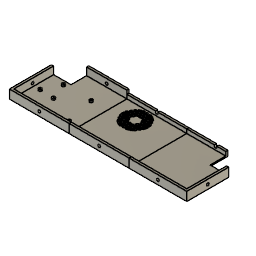
XY_Plotter_Main_Body (Autodesk Fusion 360 archive; units mm, degrees)
design "main board"
Autodesk Fusion 360 part; units mm, degrees
sketch "Sketch1" plane through (0, 0, 0) normal (0, 0, 1) x (1, 0, 0)
  line L0 (50, 35) -> (-50, 35)
  line L1 (-50, 35) -> (-50, -35)
  line L2 (-50, -35) -> (50, -35)
  line L3 (50, -35) -> (50, 35)
  line L4 (50, 35) -> (-50, -35) construction
  line L5 (-50, 35) -> (50, -35) construction
  line L6 (50, 34) -> (-50, 34) construction
  line L7 (34, -35) -> (34, 35) construction
  line L8 (-32, 35) -> (-32, -35) construction
  circle A0 centre (-30.25, 32.25) radius 1.75
  circle A1 centre (32.25, 32.25) radius 1.75
  line L9 (-49, 35) -> (-49, -35) construction
  line L10 (-50, -5) -> (50, -5) construction
  circle A2 centre (-47.25, -3.25) radius 1.75
  line L11 (-50, -34) -> (50, -34) construction
  line L12 (49, -35) -> (49, 35) construction
  circle A3 centre (47.25, -32.25) radius 1.75
  line L13 (-50, -7) -> (50, -7) construction
  line L14 (-17, 35) -> (-17, -35) construction
  circle A4 centre (-15.25, -5.25) radius 1.75
  line L15 (67.5, 67.5) -> (-67.5, 67.5)
  line L16 (-67.5, 67.5) -> (-67.5, -67.5)
  line L17 (-67.5, -67.5) -> (67.5, -67.5)
  line L18 (67.5, -67.5) -> (67.5, 67.5)
  line L19 (67.5, 67.5) -> (-67.5, -67.5) construction
  line L20 (-67.5, 67.5) -> (67.5, -67.5) construction
  dimension "d1" = 100
  dimension "d2" = 70
  dimension "d3" = -1
  dimension "d4" = -16
  dimension "d5" = -18
  dimension "d6" = 1.75
  dimension "d7" = 1.75
  dimension "d8" = -1
  dimension "d9" = -30
  dimension "d10" = 1.75
  dimension "d11" = -1
  dimension "d12" = -1
  dimension "d13" = 1.75
  dimension "d14" = -28
  dimension "d15" = -33
  dimension "d16" = 1.75
  dimension "d19" = 135
  dimension "d20" = 135
  constraint horizontal L0
  constraint perpendicular L0 L1
  constraint parallel L0 L2
  constraint parallel L1 L3
  constraint coincident L4 origin
  constraint coincident L5 origin
  constraint tangent L8 A0
  constraint tangent L6 A0
  constraint tangent L7 A1
  constraint tangent L6 A1
  constraint tangent L10 A2
  constraint tangent L9 A2
  constraint tangent L12 A3
  constraint tangent L11 A3
  constraint tangent L13 A4
  constraint tangent L14 A4
  constraint horizontal L15
  constraint perpendicular L15 L16
  constraint parallel L15 L17
  constraint parallel L16 L18
  constraint coincident L19 origin
  constraint coincident L20 origin
  measures "d1" distance of L1.end L2.end
  measures "d2" distance of L0.end L1.end
  measures "d6" radius of A0
  measures "d7" radius of A1
  measures "d10" radius of A2
  measures "d13" radius of A3
  measures "d16" radius of A4
  measures "d19" distance of L16.end L17.end
  measures "d20" distance of L15.end L16.end
extrude "Extrude1" add sketch "Sketch1" along normal blind 2 contours L0 L1 L2 L3 makes body 1
sketch "Sketch2" plane through (0, 0, 2) normal (0, 0, 1) x (-1, 0, 0)
  circle A0 centre (47.25, 3.25) radius 1.75
  circle A1 centre (30.25, -32.25) radius 1.75
  circle A2 centre (15.25, 5.25) radius 1.75
  circle A3 centre (-47.25, 32.25) radius 1.75
  circle A4 centre (-32.25, -32.25) radius 1.75
  line L0 (-50, 35) -> (-50, -35)
  line L1 (-50, -35) -> (50, -35)
  line L2 (50, -35) -> (50, 35)
  line L3 (50, 35) -> (-50, 35)
  line L4 (0, 0) -> (0, -15)
  line L5 (-67.5, -82.5) -> (67.5, -82.5)
  line L6 (67.5, -82.5) -> (67.5, 52.5)
  line L7 (67.5, 52.5) -> (-67.5, 52.5)
  line L8 (-67.5, 52.5) -> (-67.5, -82.5)
  line L9 (-67.5, -82.5) -> (67.5, 52.5) construction
  line L10 (67.5, -82.5) -> (-67.5, 52.5) construction
  line L11 (-67.5, -77.5) -> (62.5, -77.5)
  line L12 (62.5, -77.5) -> (62.5, 52.5)
  line L13 (67.5, -82.5) -> (23.5, -82.5)
  line L14 (23.5, -82.5) -> (23.5, -42.5)
  line L15 (23.5, -42.5) -> (67.5, -42.5)
  line L16 (67.5, -42.5) -> (67.5, -82.5)
  line L17 (67.5, 47.5) -> (-67.5, 47.5)
  point P0 (0, -15)
  dimension "d21" = 15
  dimension "d22" = 135
  dimension "d23" = 135
  dimension "d24" = -5
  dimension "d25" = 44
  dimension "d26" = 40
  dimension "d37" = -5
  constraint coincident L4.start origin
  constraint vertical L4
  constraint horizontal L5
  constraint perpendicular L5 L6
  constraint parallel L5 L7
  constraint parallel L6 L8
  constraint coincident L9 P0
  constraint coincident L10 P0
  constraint coincident P0 L4.end
  constraint horizontal L13
  constraint vertical L14
  constraint horizontal L15
  constraint vertical L16
  measures "d21" distance of L4.start P0
  measures "d22" distance of L6.end L7.end
  measures "d23" distance of L5.end L6.end
  measures "d25" distance of L5.end L13.end
  measures "d26" distance of L5.end L15.end
extrude "Extrude2" add sketch "Sketch2" against normal blind 3 from surface at -2 separate body contours L0 L1 L2 L3 | L5 L8 L11 L14 | L8 L11 L12 L14 L15 L17 | L7 L8 L12 L17 | L6 L12 L15 L17 | L6 L7 L12 L17 makes body 2
extrude "Extrude3" add sketch "Sketch2" along normal blind 15 and the other way blind 2 contours L5 L8 L11 L14 | L7 L8 L12 L17 | L6 L12 L15 L17 | L6 L7 L12 L17 bodies 2
sketch "Sketch3" plane through (0, 0, 0) normal (0, 0, 1) x (-1, 0, 0)
  line L0 (-67.5, -77.5) -> (23.5, -77.5)
  line L1 (23.5, -77.5) -> (23.5, -42.5)
  line L2 (23.5, -42.5) -> (62.5, -42.5)
  line L3 (62.5, -42.5) -> (62.5, 47.5)
  line L4 (62.5, 47.5) -> (-67.5, 47.5)
  line L5 (-67.5, 47.5) -> (-67.5, -77.5)
  circle A0 centre (47.25, 3.25) radius 1.75
  circle A1 centre (15.25, 5.25) radius 1.75
  circle A2 centre (30.25, -32.25) radius 1.75
  circle A3 centre (-47.25, 32.25) radius 1.75
  circle A4 centre (-32.25, -32.25) radius 1.75
  circle A5 centre (30.25, -32.25) radius 3.5
  circle A6 centre (-32.25, -32.25) radius 3.5
  circle A7 centre (-47.25, 32.25) radius 3.5
  circle A8 centre (15.25, 5.25) radius 3.5
  circle A9 centre (47.25, 3.25) radius 3.5
  circle A10 centre (15.25, 5.25) radius 1.25
  circle A11 centre (47.25, 3.25) radius 1.25
  circle A12 centre (30.25, -32.25) radius 1.25
  circle A13 centre (-32.25, -32.25) radius 1.25
  circle A14 centre (-47.25, 32.25) radius 1.25
  dimension "d38" = 7
  dimension "d39" = 7
  dimension "d40" = 7
  dimension "d41" = 7
  dimension "d42" = 7
  dimension "d43" = 2.5
  dimension "d44" = 2.5
  dimension "d45" = 2.5
  dimension "d46" = 2.5
  dimension "d47" = 2.5
  constraint concentric A2 A5
  constraint concentric A4 A6
  constraint concentric A3 A7
  constraint concentric A1 A8
  constraint concentric A0 A9
  constraint concentric A1 A10
  constraint concentric A0 A11
  constraint concentric A2 A12
  constraint concentric A4 A13
  constraint concentric A3 A14
  measures "d38" diameter of A5
  measures "d39" diameter of A6
  measures "d40" diameter of A7
  measures "d41" diameter of A8
  measures "d42" diameter of A9
  measures "d43" diameter of A10
  measures "d44" diameter of A11
  measures "d45" diameter of A12
  measures "d46" diameter of A13
  measures "d47" diameter of A14
extrude "Extrude5" add sketch "Sketch3" against normal blind 3 contours A0 | A1 | A2 | A3 | A4 bodies 2
extrude "Extrude6" add sketch "Sketch3" along normal blind 3 contours A0 | A1 | A2 | A3 | A4 | A5 | A6 | A7 | A8 | A9 bodies 2
move_body "Move1" bodies 1 to x (1, 0, 0) y (0, 1, 0) z (0, 0, 1) at (0, 0, 3)
sketch "Sketch4" plane through (0, -52.5, 0) normal (0, -1, 0) x (1, 0, 0)
  line L0 (-67.5, 17) -> (-67.5, -3)
  line L1 (-67.5, -3) -> (67.5, -3)
  line L2 (67.5, -3) -> (67.5, 17)
  line L3 (67.5, 17) -> (-67.5, 17)
  line L4 (0, 17) -> (0, -3)
  circle A0 centre (0, 7) radius 3
  circle A1 centre (0, 7) radius 4.5
  dimension "d52" = 6
  dimension "d53" = 9
  constraint midpoint L3 L4.start
  constraint midpoint L1 L4.end
  constraint midpoint L4 A0.centre
  constraint concentric A0 A1
  measures "d52" diameter of A0
  measures "d53" diameter of A1
extrude "Extrude7" cut sketch "Sketch4" against normal blind 5 contours L4 A0 | L4 A0 bodies 2
sketch "Sketch5" plane through (0, 82.5, 0) normal (0, 1, 0) x (-1, 0, 0)
  line L0 (-67.5, 17) -> (-67.5, -3)
  line L1 (-67.5, -3) -> (23.5, -3)
  line L2 (23.5, -3) -> (23.5, 17)
  line L3 (23.5, 17) -> (-67.5, 17)
  line L4 (-22, 17) -> (-22, -3) construction
  circle A0 centre (-22, 7) radius 3
  dimension "d56" = 6
  constraint midpoint L3 L4.start
  constraint midpoint L1 L4.end
  constraint midpoint L4 A0.centre
  measures "d56" diameter of A0
extrude "Extrude8" cut sketch "Sketch5" against normal blind 5 contours A0 bodies 2
sketch "Sketch6" plane through (-67.5, 0, 0) normal (-1, 0, 0) x (0, -1, 0)
  line L0 (-42.5, 17) -> (-42.5, -3)
  line L1 (-42.5, -3) -> (52.5, -3)
  line L2 (52.5, -3) -> (52.5, 17)
  line L3 (52.5, 17) -> (-42.5, 17)
  line L4 (5, 17) -> (5, -3) construction
  circle A0 centre (5, 7) radius 3
  dimension "d59" = 6
  constraint midpoint L3 L4.start
  constraint midpoint L1 L4.end
  constraint midpoint L4 A0.centre
  measures "d59" diameter of A0
extrude "Extrude9" cut sketch "Sketch6" against normal blind 5 contours A0 bodies 2
extrude "Extrude10" add 1 faces at (67.5, -50.8333, 4.6667) along direction (1, 0, 0) blind 135 separate body on bodies 2 makes body 3
extrude "Extrude11" cut 1 faces at (112.5, 79.1667, 17) along direction (0, 0, -1) blind 8 on bodies 3 bodies 3
sketch "Sketch7" plane through (0, -52.5, 0) normal (0, -1, 0) x (1, 0, 0)
  line L0 (67.5, 17) -> (67.5, -3)
  line L1 (67.5, -3) -> (202.5, -3)
  line L2 (202.5, -3) -> (202.5, 17)
  line L3 (202.5, 17) -> (67.5, 17)
  line L4 (135, 17) -> (135, -3) construction
  circle A0 centre (135, 7) radius 3
  dimension "d66" = 6
  constraint midpoint L3 L4.start
  constraint midpoint L1 L4.end
  constraint midpoint L4 A0.centre
  measures "d66" diameter of A0
extrude "Extrude12" cut sketch "Sketch7" against normal blind 135 contours A0 bodies 3
sketch "Sketch8" plane through (0, 0, -3) normal (0, 0, -1) x (1, 0, 0)
  line L0 (67.5, 52.5) -> (67.5, -82.5)
  line L1 (67.5, -82.5) -> (202.5, -82.5)
  line L2 (202.5, -82.5) -> (202.5, 52.5)
  line L3 (202.5, 52.5) -> (67.5, 52.5)
  line L4 (89.5, 52.5) -> (89.5, -82.5)
  line L5 (67.5, -74.5) -> (202.5, -74.5)
  circle A0 centre (118.5, -45.5) radius 29
  circle A1 centre (118.5, -45.5) radius 10
  line L6 (118.5, -45.5) -> (108.5, -45.5)
  line L7 (108.5, -45.5) -> (89.5, -45.5) construction
  line L8 (115.5, -47.2321) -> (118.5, -48.9641)
  line L9 (118.5, -48.9641) -> (121.5, -47.2321)
  line L10 (121.5, -47.2321) -> (121.5, -43.7679)
  line L11 (121.5, -43.7679) -> (118.5, -42.0359)
  line L12 (118.5, -42.0359) -> (115.5, -43.7679)
  line L13 (115.5, -43.7679) -> (115.5, -47.2321)
  line L14 (118.5, -45.5) -> (117, -48.0981)
  line L15 (118.5, -45.5) -> (120, -48.0981)
  line L16 (115.5, 2.9974) -> (118.5, 1.2654)
  line L17 (118.5, 1.2654) -> (121.5, 2.9974)
  line L18 (121.5, 2.9974) -> (121.5, 6.4615)
  line L19 (121.5, 6.4615) -> (118.5, 8.1936)
  line L20 (118.5, 8.1936) -> (115.5, 6.4615)
  line L21 (115.5, 6.4615) -> (115.5, 2.9974)
  line L22 (119.125, -3.2813) -> (122.125, -5.0133)
  line L23 (122.125, -5.0133) -> (125.125, -3.2813)
  line L24 (125.125, -3.2813) -> (125.125, 0.1828)
  line L25 (125.125, 0.1828) -> (122.125, 1.9149)
  line L26 (122.125, 1.9149) -> (119.125, 0.1828)
  line L27 (119.125, 0.1828) -> (119.125, -3.2813)
  line L28 (122.75, -9.5599) -> (125.75, -11.292)
  line L29 (125.75, -11.292) -> (128.75, -9.5599)
  line L30 (128.75, -9.5599) -> (128.75, -6.0958)
  line L31 (128.75, -6.0958) -> (125.75, -4.3638)
  line L32 (125.75, -4.3638) -> (122.75, -6.0958)
  line L33 (122.75, -6.0958) -> (122.75, -9.5599)
  line L34 (126.375, -15.8386) -> (129.375, -17.5707)
  line L35 (129.375, -17.5707) -> (132.375, -15.8386)
  line L36 (132.375, -15.8386) -> (132.375, -12.3745)
  line L37 (132.375, -12.3745) -> (129.375, -10.6425)
  line L38 (129.375, -10.6425) -> (126.375, -12.3745)
  line L39 (126.375, -12.3745) -> (126.375, -15.8386)
  line L40 (130, -22.1173) -> (133, -23.8494)
  line L41 (133, -23.8494) -> (136, -22.1173)
  line L42 (136, -22.1173) -> (136, -18.6532)
  line L43 (136, -18.6532) -> (133, -16.9212)
  line L44 (133, -16.9212) -> (130, -18.6532)
  line L45 (130, -18.6532) -> (130, -22.1173)
  line L46 (133.625, -28.396) -> (136.625, -30.128)
  line L47 (136.625, -30.128) -> (139.625, -28.396)
  line L48 (139.625, -28.396) -> (139.625, -24.9319)
  line L49 (139.625, -24.9319) -> (136.625, -23.1998)
  line L50 (136.625, -23.1998) -> (133.625, -24.9319)
  line L51 (133.625, -24.9319) -> (133.625, -28.396)
  line L52 (137.25, -34.6747) -> (140.25, -36.4067)
  line L53 (140.25, -36.4067) -> (143.25, -34.6747)
  line L54 (143.25, -34.6747) -> (143.25, -31.2106)
  line L55 (143.25, -31.2106) -> (140.25, -29.4785)
  line L56 (140.25, -29.4785) -> (137.25, -31.2106)
  line L57 (137.25, -31.2106) -> (137.25, -34.6747)
  line L58 (140.875, -40.9534) -> (143.875, -42.6854)
  line L59 (143.875, -42.6854) -> (146.875, -40.9534)
  line L60 (146.875, -40.9534) -> (146.875, -37.4893)
  line L61 (146.875, -37.4893) -> (143.875, -35.7572)
  line L62 (143.875, -35.7572) -> (140.875, -37.4893)
  line L63 (140.875, -37.4893) -> (140.875, -40.9534)
  line L64 (144.5, -47.2321) -> (147.5, -48.9641)
  line L65 (147.5, -48.9641) -> (150.5, -47.2321)
  line L66 (150.5, -47.2321) -> (150.5, -43.7679)
  line L67 (150.5, -43.7679) -> (147.5, -42.0359)
  line L68 (147.5, -42.0359) -> (144.5, -43.7679)
  line L69 (144.5, -43.7679) -> (144.5, -47.2321)
  line L70 (111.875, -3.2813) -> (114.875, -5.0133)
  line L71 (114.875, -5.0133) -> (117.875, -3.2813)
  line L72 (117.875, -3.2813) -> (117.875, 0.1828)
  line L73 (117.875, 0.1828) -> (114.875, 1.9149)
  line L74 (114.875, 1.9149) -> (111.875, 0.1828)
  line L75 (111.875, 0.1828) -> (111.875, -3.2813)
  line L76 (115.5, -9.5599) -> (118.5, -11.292)
  line L77 (118.5, -11.292) -> (121.5, -9.5599)
  line L78 (121.5, -9.5599) -> (121.5, -6.0958)
  line L79 (121.5, -6.0958) -> (118.5, -4.3638)
  line L80 (118.5, -4.3638) -> (115.5, -6.0958)
  line L81 (115.5, -6.0958) -> (115.5, -9.5599)
  line L82 (119.125, -15.8386) -> (122.125, -17.5707)
  line L83 (122.125, -17.5707) -> (125.125, -15.8386)
  line L84 (125.125, -15.8386) -> (125.125, -12.3745)
  line L85 (125.125, -12.3745) -> (122.125, -10.6425)
  line L86 (122.125, -10.6425) -> (119.125, -12.3745)
  line L87 (119.125, -12.3745) -> (119.125, -15.8386)
  line L88 (122.75, -22.1173) -> (125.75, -23.8494)
  line L89 (125.75, -23.8494) -> (128.75, -22.1173)
  line L90 (128.75, -22.1173) -> (128.75, -18.6532)
  line L91 (128.75, -18.6532) -> (125.75, -16.9212)
  line L92 (125.75, -16.9212) -> (122.75, -18.6532)
  line L93 (122.75, -18.6532) -> (122.75, -22.1173)
  line L94 (126.375, -28.396) -> (129.375, -30.128)
  line L95 (129.375, -30.128) -> (132.375, -28.396)
  line L96 (132.375, -28.396) -> (132.375, -24.9319)
  line L97 (132.375, -24.9319) -> (129.375, -23.1998)
  line L98 (129.375, -23.1998) -> (126.375, -24.9319)
  line L99 (126.375, -24.9319) -> (126.375, -28.396)
  line L100 (130, -34.6747) -> (133, -36.4067)
  line L101 (133, -36.4067) -> (136, -34.6747)
  line L102 (136, -34.6747) -> (136, -31.2106)
  line L103 (136, -31.2106) -> (133, -29.4785)
  line L104 (133, -29.4785) -> (130, -31.2106)
  line L105 (130, -31.2106) -> (130, -34.6747)
  line L106 (133.625, -40.9534) -> (136.625, -42.6854)
  line L107 (136.625, -42.6854) -> (139.625, -40.9534)
  line L108 (139.625, -40.9534) -> (139.625, -37.4893)
  line L109 (139.625, -37.4893) -> (136.625, -35.7572)
  line L110 (136.625, -35.7572) -> (133.625, -37.4893)
  line L111 (133.625, -37.4893) -> (133.625, -40.9534)
  line L112 (137.25, -47.2321) -> (140.25, -48.9641)
  line L113 (140.25, -48.9641) -> (143.25, -47.2321)
  line L114 (143.25, -47.2321) -> (143.25, -43.7679)
  line L115 (143.25, -43.7679) -> (140.25, -42.0359)
  line L116 (140.25, -42.0359) -> (137.25, -43.7679)
  line L117 (137.25, -43.7679) -> (137.25, -47.2321)
  line L118 (140.875, -53.5107) -> (143.875, -55.2428)
  line L119 (143.875, -55.2428) -> (146.875, -53.5107)
  line L120 (146.875, -53.5107) -> (146.875, -50.0466)
  line L121 (146.875, -50.0466) -> (143.875, -48.3146)
  line L122 (143.875, -48.3146) -> (140.875, -50.0466)
  line L123 (140.875, -50.0466) -> (140.875, -53.5107)
  line L124 (108.25, -9.5599) -> (111.25, -11.292)
  line L125 (111.25, -11.292) -> (114.25, -9.5599)
  line L126 (114.25, -9.5599) -> (114.25, -6.0958)
  line L127 (114.25, -6.0958) -> (111.25, -4.3638)
  line L128 (111.25, -4.3638) -> (108.25, -6.0958)
  line L129 (108.25, -6.0958) -> (108.25, -9.5599)
  line L130 (111.875, -15.8386) -> (114.875, -17.5707)
  line L131 (114.875, -17.5707) -> (117.875, -15.8386)
  line L132 (117.875, -15.8386) -> (117.875, -12.3745)
  line L133 (117.875, -12.3745) -> (114.875, -10.6425)
  line L134 (114.875, -10.6425) -> (111.875, -12.3745)
  line L135 (111.875, -12.3745) -> (111.875, -15.8386)
  line L136 (115.5, -22.1173) -> (118.5, -23.8494)
  line L137 (118.5, -23.8494) -> (121.5, -22.1173)
  line L138 (121.5, -22.1173) -> (121.5, -18.6532)
  line L139 (121.5, -18.6532) -> (118.5, -16.9212)
  line L140 (118.5, -16.9212) -> (115.5, -18.6532)
  line L141 (115.5, -18.6532) -> (115.5, -22.1173)
  line L142 (119.125, -28.396) -> (122.125, -30.128)
  line L143 (122.125, -30.128) -> (125.125, -28.396)
  line L144 (125.125, -28.396) -> (125.125, -24.9319)
  line L145 (125.125, -24.9319) -> (122.125, -23.1998)
  line L146 (122.125, -23.1998) -> (119.125, -24.9319)
  line L147 (119.125, -24.9319) -> (119.125, -28.396)
  line L148 (122.75, -34.6747) -> (125.75, -36.4067)
  line L149 (125.75, -36.4067) -> (128.75, -34.6747)
  line L150 (128.75, -34.6747) -> (128.75, -31.2106)
  line L151 (128.75, -31.2106) -> (125.75, -29.4785)
  line L152 (125.75, -29.4785) -> (122.75, -31.2106)
  line L153 (122.75, -31.2106) -> (122.75, -34.6747)
  line L154 (126.375, -40.9534) -> (129.375, -42.6854)
  line L155 (129.375, -42.6854) -> (132.375, -40.9534)
  line L156 (132.375, -40.9534) -> (132.375, -37.4893)
  line L157 (132.375, -37.4893) -> (129.375, -35.7572)
  line L158 (129.375, -35.7572) -> (126.375, -37.4893)
  line L159 (126.375, -37.4893) -> (126.375, -40.9534)
  line L160 (130, -47.2321) -> (133, -48.9641)
  line L161 (133, -48.9641) -> (136, -47.2321)
  line L162 (136, -47.2321) -> (136, -43.7679)
  line L163 (136, -43.7679) -> (133, -42.0359)
  line L164 (133, -42.0359) -> (130, -43.7679)
  line L165 (130, -43.7679) -> (130, -47.2321)
  line L166 (133.625, -53.5107) -> (136.625, -55.2428)
  line L167 (136.625, -55.2428) -> (139.625, -53.5107)
  line L168 (139.625, -53.5107) -> (139.625, -50.0466)
  line L169 (139.625, -50.0466) -> (136.625, -48.3146)
  line L170 (136.625, -48.3146) -> (133.625, -50.0466)
  line L171 (133.625, -50.0466) -> (133.625, -53.5107)
  line L172 (137.25, -59.7894) -> (140.25, -61.5215)
  line L173 (140.25, -61.5215) -> (143.25, -59.7894)
  line L174 (143.25, -59.7894) -> (143.25, -56.3253)
  line L175 (143.25, -56.3253) -> (140.25, -54.5933)
  line L176 (140.25, -54.5933) -> (137.25, -56.3253)
  line L177 (137.25, -56.3253) -> (137.25, -59.7894)
  line L178 (104.625, -15.8386) -> (107.625, -17.5707)
  line L179 (107.625, -17.5707) -> (110.625, -15.8386)
  line L180 (110.625, -15.8386) -> (110.625, -12.3745)
  line L181 (110.625, -12.3745) -> (107.625, -10.6425)
  line L182 (107.625, -10.6425) -> (104.625, -12.3745)
  line L183 (104.625, -12.3745) -> (104.625, -15.8386)
  line L184 (108.25, -22.1173) -> (111.25, -23.8494)
  line L185 (111.25, -23.8494) -> (114.25, -22.1173)
  line L186 (114.25, -22.1173) -> (114.25, -18.6532)
  line L187 (114.25, -18.6532) -> (111.25, -16.9212)
  line L188 (111.25, -16.9212) -> (108.25, -18.6532)
  line L189 (108.25, -18.6532) -> (108.25, -22.1173)
  line L190 (111.875, -28.396) -> (114.875, -30.128)
  line L191 (114.875, -30.128) -> (117.875, -28.396)
  line L192 (117.875, -28.396) -> (117.875, -24.9319)
  line L193 (117.875, -24.9319) -> (114.875, -23.1998)
  line L194 (114.875, -23.1998) -> (111.875, -24.9319)
  line L195 (111.875, -24.9319) -> (111.875, -28.396)
  line L196 (115.5, -34.6747) -> (118.5, -36.4067)
  line L197 (118.5, -36.4067) -> (121.5, -34.6747)
  line L198 (121.5, -34.6747) -> (121.5, -31.2106)
  line L199 (121.5, -31.2106) -> (118.5, -29.4785)
  line L200 (118.5, -29.4785) -> (115.5, -31.2106)
  line L201 (115.5, -31.2106) -> (115.5, -34.6747)
  line L202 (119.125, -40.9534) -> (122.125, -42.6854)
  line L203 (122.125, -42.6854) -> (125.125, -40.9534)
  line L204 (125.125, -40.9534) -> (125.125, -37.4893)
  line L205 (125.125, -37.4893) -> (122.125, -35.7572)
  line L206 (122.125, -35.7572) -> (119.125, -37.4893)
  line L207 (119.125, -37.4893) -> (119.125, -40.9534)
  line L208 (122.75, -47.2321) -> (125.75, -48.9641)
  line L209 (125.75, -48.9641) -> (128.75, -47.2321)
  line L210 (128.75, -47.2321) -> (128.75, -43.7679)
  line L211 (128.75, -43.7679) -> (125.75, -42.0359)
  line L212 (125.75, -42.0359) -> (122.75, -43.7679)
  line L213 (122.75, -43.7679) -> (122.75, -47.2321)
  line L214 (126.375, -53.5107) -> (129.375, -55.2428)
  line L215 (129.375, -55.2428) -> (132.375, -53.5107)
  line L216 (132.375, -53.5107) -> (132.375, -50.0466)
  line L217 (132.375, -50.0466) -> (129.375, -48.3146)
  line L218 (129.375, -48.3146) -> (126.375, -50.0466)
  line L219 (126.375, -50.0466) -> (126.375, -53.5107)
  line L220 (130, -59.7894) -> (133, -61.5215)
  line L221 (133, -61.5215) -> (136, -59.7894)
  line L222 (136, -59.7894) -> (136, -56.3253)
  line L223 (136, -56.3253) -> (133, -54.5933)
  line L224 (133, -54.5933) -> (130, -56.3253)
  line L225 (130, -56.3253) -> (130, -59.7894)
  line L226 (133.625, -66.0681) -> (136.625, -67.8002)
  line L227 (136.625, -67.8002) -> (139.625, -66.0681)
  line L228 (139.625, -66.0681) -> (139.625, -62.604)
  line L229 (139.625, -62.604) -> (136.625, -60.872)
  line L230 (136.625, -60.872) -> (133.625, -62.604)
  line L231 (133.625, -62.604) -> (133.625, -66.0681)
  line L232 (101, -22.1173) -> (104, -23.8494)
  line L233 (104, -23.8494) -> (107, -22.1173)
  line L234 (107, -22.1173) -> (107, -18.6532)
  line L235 (107, -18.6532) -> (104, -16.9212)
  line L236 (104, -16.9212) -> (101, -18.6532)
  line L237 (101, -18.6532) -> (101, -22.1173)
  line L238 (104.625, -28.396) -> (107.625, -30.128)
  line L239 (107.625, -30.128) -> (110.625, -28.396)
  line L240 (110.625, -28.396) -> (110.625, -24.9319)
  line L241 (110.625, -24.9319) -> (107.625, -23.1998)
  line L242 (107.625, -23.1998) -> (104.625, -24.9319)
  line L243 (104.625, -24.9319) -> (104.625, -28.396)
  line L244 (108.25, -34.6747) -> (111.25, -36.4067)
  line L245 (111.25, -36.4067) -> (114.25, -34.6747)
  line L246 (114.25, -34.6747) -> (114.25, -31.2106)
  line L247 (114.25, -31.2106) -> (111.25, -29.4785)
  line L248 (111.25, -29.4785) -> (108.25, -31.2106)
  line L249 (108.25, -31.2106) -> (108.25, -34.6747)
  line L250 (111.875, -40.9534) -> (114.875, -42.6854)
  line L251 (114.875, -42.6854) -> (117.875, -40.9534)
  line L252 (117.875, -40.9534) -> (117.875, -37.4893)
  line L253 (117.875, -37.4893) -> (114.875, -35.7572)
  line L254 (114.875, -35.7572) -> (111.875, -37.4893)
  line L255 (111.875, -37.4893) -> (111.875, -40.9534)
  line L256 (119.125, -53.5107) -> (122.125, -55.2428)
  line L257 (122.125, -55.2428) -> (125.125, -53.5107)
  line L258 (125.125, -53.5107) -> (125.125, -50.0466)
  line L259 (125.125, -50.0466) -> (122.125, -48.3146)
  line L260 (122.125, -48.3146) -> (119.125, -50.0466)
  line L261 (119.125, -50.0466) -> (119.125, -53.5107)
  line L262 (122.75, -59.7894) -> (125.75, -61.5215)
  line L263 (125.75, -61.5215) -> (128.75, -59.7894)
  line L264 (128.75, -59.7894) -> (128.75, -56.3253)
  line L265 (128.75, -56.3253) -> (125.75, -54.5933)
  line L266 (125.75, -54.5933) -> (122.75, -56.3253)
  line L267 (122.75, -56.3253) -> (122.75, -59.7894)
  line L268 (126.375, -66.0681) -> (129.375, -67.8002)
  line L269 (129.375, -67.8002) -> (132.375, -66.0681)
  line L270 (132.375, -66.0681) -> (132.375, -62.604)
  line L271 (132.375, -62.604) -> (129.375, -60.872)
  line L272 (129.375, -60.872) -> (126.375, -62.604)
  line L273 (126.375, -62.604) -> (126.375, -66.0681)
  line L274 (130, -72.3468) -> (133, -74.0788)
  line L275 (133, -74.0788) -> (136, -72.3468)
  line L276 (136, -72.3468) -> (136, -68.8827)
  line L277 (136, -68.8827) -> (133, -67.1506)
  line L278 (133, -67.1506) -> (130, -68.8827)
  line L279 (130, -68.8827) -> (130, -72.3468)
  line L280 (97.375, -28.396) -> (100.375, -30.128)
  line L281 (100.375, -30.128) -> (103.375, -28.396)
  line L282 (103.375, -28.396) -> (103.375, -24.9319)
  line L283 (103.375, -24.9319) -> (100.375, -23.1998)
  line L284 (100.375, -23.1998) -> (97.375, -24.9319)
  line L285 (97.375, -24.9319) -> (97.375, -28.396)
  line L286 (101, -34.6747) -> (104, -36.4067)
  line L287 (104, -36.4067) -> (107, -34.6747)
  line L288 (107, -34.6747) -> (107, -31.2106)
  line L289 (107, -31.2106) -> (104, -29.4785)
  line L290 (104, -29.4785) -> (101, -31.2106)
  line L291 (101, -31.2106) -> (101, -34.6747)
  line L292 (104.625, -40.9534) -> (107.625, -42.6854)
  line L293 (107.625, -42.6854) -> (110.625, -40.9534)
  line L294 (110.625, -40.9534) -> (110.625, -37.4893)
  line L295 (110.625, -37.4893) -> (107.625, -35.7572)
  line L296 (107.625, -35.7572) -> (104.625, -37.4893)
  line L297 (104.625, -37.4893) -> (104.625, -40.9534)
  line L298 (108.25, -47.2321) -> (111.25, -48.9641)
  line L299 (111.25, -48.9641) -> (114.25, -47.2321)
  line L300 (114.25, -47.2321) -> (114.25, -43.7679)
  line L301 (114.25, -43.7679) -> (111.25, -42.0359)
  line L302 (111.25, -42.0359) -> (108.25, -43.7679)
  line L303 (108.25, -43.7679) -> (108.25, -47.2321)
  line L304 (111.875, -53.5107) -> (114.875, -55.2428)
  line L305 (114.875, -55.2428) -> (117.875, -53.5107)
  line L306 (117.875, -53.5107) -> (117.875, -50.0466)
  line L307 (117.875, -50.0466) -> (114.875, -48.3146)
  line L308 (114.875, -48.3146) -> (111.875, -50.0466)
  line L309 (111.875, -50.0466) -> (111.875, -53.5107)
  line L310 (115.5, -59.7894) -> (118.5, -61.5215)
  line L311 (118.5, -61.5215) -> (121.5, -59.7894)
  line L312 (121.5, -59.7894) -> (121.5, -56.3253)
  line L313 (121.5, -56.3253) -> (118.5, -54.5933)
  line L314 (118.5, -54.5933) -> (115.5, -56.3253)
  line L315 (115.5, -56.3253) -> (115.5, -59.7894)
  line L316 (119.125, -66.0681) -> (122.125, -67.8002)
  line L317 (122.125, -67.8002) -> (125.125, -66.0681)
  line L318 (125.125, -66.0681) -> (125.125, -62.604)
  line L319 (125.125, -62.604) -> (122.125, -60.872)
  line L320 (122.125, -60.872) -> (119.125, -62.604)
  line L321 (119.125, -62.604) -> (119.125, -66.0681)
  line L322 (122.75, -72.3468) -> (125.75, -74.0788)
  line L323 (125.75, -74.0788) -> (128.75, -72.3468)
  line L324 (128.75, -72.3468) -> (128.75, -68.8827)
  line L325 (128.75, -68.8827) -> (125.75, -67.1506)
  line L326 (125.75, -67.1506) -> (122.75, -68.8827)
  line L327 (122.75, -68.8827) -> (122.75, -72.3468)
  line L328 (126.375, -78.6255) -> (129.375, -80.3575)
  line L329 (129.375, -80.3575) -> (132.375, -78.6255)
  line L330 (132.375, -78.6255) -> (132.375, -75.1614)
  line L331 (132.375, -75.1614) -> (129.375, -73.4293)
  line L332 (129.375, -73.4293) -> (126.375, -75.1614)
  line L333 (126.375, -75.1614) -> (126.375, -78.6255)
  line L334 (93.75, -34.6747) -> (96.75, -36.4067)
  line L335 (96.75, -36.4067) -> (99.75, -34.6747)
  line L336 (99.75, -34.6747) -> (99.75, -31.2106)
  line L337 (99.75, -31.2106) -> (96.75, -29.4785)
  line L338 (96.75, -29.4785) -> (93.75, -31.2106)
  line L339 (93.75, -31.2106) -> (93.75, -34.6747)
  line L340 (97.375, -40.9534) -> (100.375, -42.6854)
  line L341 (100.375, -42.6854) -> (103.375, -40.9534)
  line L342 (103.375, -40.9534) -> (103.375, -37.4893)
  line L343 (103.375, -37.4893) -> (100.375, -35.7572)
  line L344 (100.375, -35.7572) -> (97.375, -37.4893)
  line L345 (97.375, -37.4893) -> (97.375, -40.9534)
  line L346 (101, -47.2321) -> (104, -48.9641)
  line L347 (104, -48.9641) -> (107, -47.2321)
  line L348 (107, -47.2321) -> (107, -43.7679)
  line L349 (107, -43.7679) -> (104, -42.0359)
  line L350 (104, -42.0359) -> (101, -43.7679)
  line L351 (101, -43.7679) -> (101, -47.2321)
  line L352 (104.625, -53.5107) -> (107.625, -55.2428)
  line L353 (107.625, -55.2428) -> (110.625, -53.5107)
  line L354 (110.625, -53.5107) -> (110.625, -50.0466)
  line L355 (110.625, -50.0466) -> (107.625, -48.3146)
  line L356 (107.625, -48.3146) -> (104.625, -50.0466)
  line L357 (104.625, -50.0466) -> (104.625, -53.5107)
  line L358 (108.25, -59.7894) -> (111.25, -61.5215)
  line L359 (111.25, -61.5215) -> (114.25, -59.7894)
  line L360 (114.25, -59.7894) -> (114.25, -56.3253)
  line L361 (114.25, -56.3253) -> (111.25, -54.5933)
  line L362 (111.25, -54.5933) -> (108.25, -56.3253)
  line L363 (108.25, -56.3253) -> (108.25, -59.7894)
  line L364 (111.875, -66.0681) -> (114.875, -67.8002)
  line L365 (114.875, -67.8002) -> (117.875, -66.0681)
  line L366 (117.875, -66.0681) -> (117.875, -62.604)
  line L367 (117.875, -62.604) -> (114.875, -60.872)
  line L368 (114.875, -60.872) -> (111.875, -62.604)
  line L369 (111.875, -62.604) -> (111.875, -66.0681)
  line L370 (115.5, -72.3468) -> (118.5, -74.0788)
  line L371 (118.5, -74.0788) -> (121.5, -72.3468)
  line L372 (121.5, -72.3468) -> (121.5, -68.8827)
  line L373 (121.5, -68.8827) -> (118.5, -67.1506)
  line L374 (118.5, -67.1506) -> (115.5, -68.8827)
  line L375 (115.5, -68.8827) -> (115.5, -72.3468)
  line L376 (119.125, -78.6255) -> (122.125, -80.3575)
  line L377 (122.125, -80.3575) -> (125.125, -78.6255)
  line L378 (125.125, -78.6255) -> (125.125, -75.1614)
  line L379 (125.125, -75.1614) -> (122.125, -73.4293)
  line L380 (122.125, -73.4293) -> (119.125, -75.1614)
  line L381 (119.125, -75.1614) -> (119.125, -78.6255)
  line L382 (122.75, -84.9042) -> (125.75, -86.6362)
  line L383 (125.75, -86.6362) -> (128.75, -84.9042)
  line L384 (128.75, -84.9042) -> (128.75, -81.4401)
  line L385 (128.75, -81.4401) -> (125.75, -79.708)
  line L386 (125.75, -79.708) -> (122.75, -81.4401)
  line L387 (122.75, -81.4401) -> (122.75, -84.9042)
  line L388 (90.125, -40.9534) -> (93.125, -42.6854)
  line L389 (93.125, -42.6854) -> (96.125, -40.9534)
  line L390 (96.125, -40.9534) -> (96.125, -37.4893)
  line L391 (96.125, -37.4893) -> (93.125, -35.7572)
  line L392 (93.125, -35.7572) -> (90.125, -37.4893)
  line L393 (90.125, -37.4893) -> (90.125, -40.9534)
  line L394 (93.75, -47.2321) -> (96.75, -48.9641)
  line L395 (96.75, -48.9641) -> (99.75, -47.2321)
  line L396 (99.75, -47.2321) -> (99.75, -43.7679)
  line L397 (99.75, -43.7679) -> (96.75, -42.0359)
  line L398 (96.75, -42.0359) -> (93.75, -43.7679)
  line L399 (93.75, -43.7679) -> (93.75, -47.2321)
  line L400 (97.375, -53.5107) -> (100.375, -55.2428)
  line L401 (100.375, -55.2428) -> (103.375, -53.5107)
  line L402 (103.375, -53.5107) -> (103.375, -50.0466)
  line L403 (103.375, -50.0466) -> (100.375, -48.3146)
  line L404 (100.375, -48.3146) -> (97.375, -50.0466)
  line L405 (97.375, -50.0466) -> (97.375, -53.5107)
  line L406 (101, -59.7894) -> (104, -61.5215)
  line L407 (104, -61.5215) -> (107, -59.7894)
  line L408 (107, -59.7894) -> (107, -56.3253)
  line L409 (107, -56.3253) -> (104, -54.5933)
  line L410 (104, -54.5933) -> (101, -56.3253)
  line L411 (101, -56.3253) -> (101, -59.7894)
  line L412 (104.625, -66.0681) -> (107.625, -67.8002)
  line L413 (107.625, -67.8002) -> (110.625, -66.0681)
  line L414 (110.625, -66.0681) -> (110.625, -62.604)
  line L415 (110.625, -62.604) -> (107.625, -60.872)
  line L416 (107.625, -60.872) -> (104.625, -62.604)
  line L417 (104.625, -62.604) -> (104.625, -66.0681)
  line L418 (108.25, -72.3468) -> (111.25, -74.0788)
  line L419 (111.25, -74.0788) -> (114.25, -72.3468)
  line L420 (114.25, -72.3468) -> (114.25, -68.8827)
  line L421 (114.25, -68.8827) -> (111.25, -67.1506)
  line L422 (111.25, -67.1506) -> (108.25, -68.8827)
  line L423 (108.25, -68.8827) -> (108.25, -72.3468)
  line L424 (111.875, -78.6255) -> (114.875, -80.3575)
  line L425 (114.875, -80.3575) -> (117.875, -78.6255)
  line L426 (117.875, -78.6255) -> (117.875, -75.1614)
  line L427 (117.875, -75.1614) -> (114.875, -73.4293)
  line L428 (114.875, -73.4293) -> (111.875, -75.1614)
  line L429 (111.875, -75.1614) -> (111.875, -78.6255)
  line L430 (115.5, -84.9042) -> (118.5, -86.6362)
  line L431 (118.5, -86.6362) -> (121.5, -84.9042)
  line L432 (121.5, -84.9042) -> (121.5, -81.4401)
  line L433 (121.5, -81.4401) -> (118.5, -79.708)
  line L434 (118.5, -79.708) -> (115.5, -81.4401)
  line L435 (115.5, -81.4401) -> (115.5, -84.9042)
  line L436 (119.125, -91.1828) -> (122.125, -92.9149)
  line L437 (122.125, -92.9149) -> (125.125, -91.1828)
  line L438 (125.125, -91.1828) -> (125.125, -87.7187)
  line L439 (125.125, -87.7187) -> (122.125, -85.9867)
  line L440 (122.125, -85.9867) -> (119.125, -87.7187)
  line L441 (119.125, -87.7187) -> (119.125, -91.1828)
  line L442 (86.5, -47.2321) -> (89.5, -48.9641)
  line L443 (89.5, -48.9641) -> (92.5, -47.2321)
  line L444 (92.5, -47.2321) -> (92.5, -43.7679)
  line L445 (92.5, -43.7679) -> (89.5, -42.0359)
  line L446 (89.5, -42.0359) -> (86.5, -43.7679)
  line L447 (86.5, -43.7679) -> (86.5, -47.2321)
  line L448 (90.125, -53.5107) -> (93.125, -55.2428)
  line L449 (93.125, -55.2428) -> (96.125, -53.5107)
  line L450 (96.125, -53.5107) -> (96.125, -50.0466)
  line L451 (96.125, -50.0466) -> (93.125, -48.3146)
  line L452 (93.125, -48.3146) -> (90.125, -50.0466)
  line L453 (90.125, -50.0466) -> (90.125, -53.5107)
  line L454 (93.75, -59.7894) -> (96.75, -61.5215)
  line L455 (96.75, -61.5215) -> (99.75, -59.7894)
  line L456 (99.75, -59.7894) -> (99.75, -56.3253)
  line L457 (99.75, -56.3253) -> (96.75, -54.5933)
  line L458 (96.75, -54.5933) -> (93.75, -56.3253)
  line L459 (93.75, -56.3253) -> (93.75, -59.7894)
  line L460 (97.375, -66.0681) -> (100.375, -67.8002)
  line L461 (100.375, -67.8002) -> (103.375, -66.0681)
  line L462 (103.375, -66.0681) -> (103.375, -62.604)
  line L463 (103.375, -62.604) -> (100.375, -60.872)
  line L464 (100.375, -60.872) -> (97.375, -62.604)
  line L465 (97.375, -62.604) -> (97.375, -66.0681)
  line L466 (101, -72.3468) -> (104, -74.0788)
  line L467 (104, -74.0788) -> (107, -72.3468)
  line L468 (107, -72.3468) -> (107, -68.8827)
  line L469 (107, -68.8827) -> (104, -67.1506)
  line L470 (104, -67.1506) -> (101, -68.8827)
  line L471 (101, -68.8827) -> (101, -72.3468)
  line L472 (104.625, -78.6255) -> (107.625, -80.3575)
  line L473 (107.625, -80.3575) -> (110.625, -78.6255)
  line L474 (110.625, -78.6255) -> (110.625, -75.1614)
  line L475 (110.625, -75.1614) -> (107.625, -73.4293)
  line L476 (107.625, -73.4293) -> (104.625, -75.1614)
  line L477 (104.625, -75.1614) -> (104.625, -78.6255)
  line L478 (108.25, -84.9042) -> (111.25, -86.6362)
  line L479 (111.25, -86.6362) -> (114.25, -84.9042)
  line L480 (114.25, -84.9042) -> (114.25, -81.4401)
  line L481 (114.25, -81.4401) -> (111.25, -79.708)
  line L482 (111.25, -79.708) -> (108.25, -81.4401)
  line L483 (108.25, -81.4401) -> (108.25, -84.9042)
  line L484 (111.875, -91.1828) -> (114.875, -92.9149)
  line L485 (114.875, -92.9149) -> (117.875, -91.1828)
  line L486 (117.875, -91.1828) -> (117.875, -87.7187)
  line L487 (117.875, -87.7187) -> (114.875, -85.9867)
  line L488 (114.875, -85.9867) -> (111.875, -87.7187)
  line L489 (111.875, -87.7187) -> (111.875, -91.1828)
  line L490 (115.5, -97.4615) -> (118.5, -99.1936)
  line L491 (118.5, -99.1936) -> (121.5, -97.4615)
  line L492 (121.5, -97.4615) -> (121.5, -93.9974)
  line L493 (121.5, -93.9974) -> (118.5, -92.2654)
  line L494 (118.5, -92.2654) -> (115.5, -93.9974)
  line L495 (115.5, -93.9974) -> (115.5, -97.4615)
  point P0 (118.5, -45.5)
  point P1 (120, 2.1314)
  point P2 (123.625, -4.1473)
  point P3 (127.25, -10.426)
  point P4 (130.875, -16.7047)
  point P5 (134.5, -22.9833)
  point P6 (138.125, -29.262)
  point P7 (141.75, -35.5407)
  point P8 (145.375, -41.8194)
  point P9 (149, -48.0981)
  point P10 (116.375, -4.1473)
  point P11 (120, -10.426)
  point P12 (123.625, -16.7047)
  point P13 (127.25, -22.9833)
  point P14 (130.875, -29.262)
  point P15 (134.5, -35.5407)
  point P16 (138.125, -41.8194)
  point P17 (141.75, -48.0981)
  point P18 (145.375, -54.3768)
  point P19 (112.75, -10.426)
  point P20 (116.375, -16.7047)
  point P21 (120, -22.9833)
  point P22 (123.625, -29.262)
  point P23 (127.25, -35.5407)
  point P24 (130.875, -41.8194)
  point P25 (134.5, -48.0981)
  point P26 (138.125, -54.3768)
  point P27 (141.75, -60.6554)
  point P28 (109.125, -16.7047)
  point P29 (112.75, -22.9833)
  point P30 (116.375, -29.262)
  point P31 (120, -35.5407)
  point P32 (123.625, -41.8194)
  point P33 (127.25, -48.0981)
  point P34 (130.875, -54.3768)
  point P35 (134.5, -60.6554)
  point P36 (138.125, -66.9341)
  point P37 (105.5, -22.9833)
  point P38 (109.125, -29.262)
  point P39 (112.75, -35.5407)
  point P40 (116.375, -41.8194)
  point P41 (123.625, -54.3768)
  point P42 (127.25, -60.6554)
  point P43 (130.875, -66.9341)
  point P44 (134.5, -73.2128)
  point P45 (101.875, -29.262)
  point P46 (105.5, -35.5407)
  point P47 (109.125, -41.8194)
  point P48 (112.75, -48.0981)
  point P49 (116.375, -54.3768)
  point P50 (120, -60.6554)
  point P51 (123.625, -66.9341)
  point P52 (127.25, -73.2128)
  point P53 (130.875, -79.4915)
  point P54 (98.25, -35.5407)
  point P55 (101.875, -41.8194)
  point P56 (105.5, -48.0981)
  point P57 (109.125, -54.3768)
  point P58 (112.75, -60.6554)
  point P59 (116.375, -66.9341)
  point P60 (120, -73.2128)
  point P61 (123.625, -79.4915)
  point P62 (127.25, -85.7702)
  point P63 (94.625, -41.8194)
  point P64 (98.25, -48.0981)
  point P65 (101.875, -54.3768)
  point P66 (105.5, -60.6554)
  point P67 (109.125, -66.9341)
  point P68 (112.75, -73.2128)
  point P69 (116.375, -79.4915)
  point P70 (120, -85.7702)
  point P71 (123.625, -92.0489)
  point P72 (91, -48.0981)
  point P73 (94.625, -54.3768)
  point P74 (98.25, -60.6554)
  point P75 (101.875, -66.9341)
  point P76 (105.5, -73.2128)
  point P77 (109.125, -79.4915)
  point P78 (112.75, -85.7702)
  point P79 (116.375, -92.0489)
  point P80 (120, -98.3275)
  dimension "d69" = -22
  dimension "d70" = -8
  dimension "d71" = 29
  dimension "d72" = 20
  dimension "d73" = 3
  dimension "d76" = 29
  dimension "d77" = 29
  constraint tangent L5 A0
  constraint tangent L4 A0
  constraint concentric A0 A1
  constraint coincident P0 A0.centre
  constraint coincident A1 L6.end
  constraint horizontal L6
  constraint coincident A0 L7.end
  constraint perpendicular L4 L7
  constraint midpoint L8 L14.end
  constraint midpoint L9 L15.end
  measures "d71" radius of A0
  measures "d72" diameter of A1
  measures "d73" distance of P0 L13
extrude "Extrude13" cut sketch "Sketch8" against normal blind 3 contours A0 L443 L444 L445 | A0 L388 L389 L390 L391 L392 L393 | A0 L448 L449 L450 L451 L452 L453 | A0 L280 L281 L282 L283 L284 L285 | A0 L460 L461 L462 L463 L464 L465 | A0 L418 L419 L420 L421 L422 L423 | A0 L322 L323 L324 L325 L326 L327 | A0 L232 L233 L234 | A0 L468 L469 L470 | A0 L277 L278 L279 | A0 L184 L185 L186 L187 L188 L189 | A0 L226 L227 L228 L229 L230 L231 | A0 L118 L119 L120 L121 L122 L123 | A0 L64 L68 L69 | A0 L88 L89 L90 L91 L92 L93 | A0 L40 L41 L45 | A0 L58 L59 L60 L61 L62 L63 | A0 L46 L47 L48 L49 L50 L51 | A1 L154 L155 L156 L157 L158 L159 | A1 L214 L215 L216 L217 L218 L219 | A1 L196 L197 L198 L199 L200 L201 | A1 L310 L311 L312 L313 L314 L315 | A1 L292 L293 L294 L295 L296 L297 | A1 L352 L353 L354 L355 L356 L357 | L52 L53 L54 L55 L56 L57 | L94 L95 L96 L97 L98 L99 | L100 L101 L102 L103 L104 L105 | L106 L107 L108 L109 L110 L111 | L112 L113 L114 L115 L116 L117 | L136 L137 L138 L139 L140 L141 | L142 L143 L144 L145 L146 L147 | L148 L149 L150 L151 L152 L153 | L160 L161 L162 L163 L164 L165 | L166 L167 L168 L169 L170 L171 | L172 L173 L174 L175 L176 L177 | L190 L191 L192 L193 L194 L195 | L220 L221 L222 L223 L224 L225 | L238 L239 L240 L241 L242 L243 | L244 L245 L246 L247 L248 L249 | L262 L263 L264 L265 L266 L267 | L268 L269 L270 L271 L272 L273 | L286 L287 L288 L289 L290 L291 | L316 L317 L318 L319 L320 L321 | L334 L335 L336 L337 L338 L339 | L340 L341 L342 L343 L344 L345 | L346 L347 L348 L349 L350 L351 | L358 L359 L360 L361 L362 L363 | L364 L365 L366 L367 L368 L369 | L370 L371 L372 L373 L374 L375 | L394 L395 L396 L397 L398 L399 | L400 L401 L402 L403 L404 L405 | L406 L407 L408 L409 L410 L411 | L412 L413 L414 L415 L416 L417 | L454 L455 L456 L457 L458 L459 bodies 3
extrude "Extrude14" add 1 faces at (202.5, -50.8333, 4.6667) along direction (1, 0, 0) blind 130 separate body on bodies 3 makes body 4
sketch "Sketch9" plane through (0, 0, -3) normal (0, 0, -1) x (1, 0, 0)
  line L0 (202.5, 52.5) -> (202.5, -82.5)
  line L1 (202.5, -82.5) -> (332.5, -82.5)
  line L2 (332.5, -82.5) -> (332.5, 52.5)
  line L3 (332.5, 52.5) -> (202.5, 52.5)
  line L4 (332.5, -82.5) -> (290.5, -82.5)
  line L5 (290.5, -82.5) -> (290.5, -42.5)
  line L6 (290.5, -42.5) -> (332.5, -42.5)
  line L7 (332.5, -42.5) -> (332.5, -82.5)
  dimension "d82" = 42
  dimension "d83" = 40
  constraint horizontal L4
  constraint vertical L5
  constraint horizontal L6
  constraint vertical L7
  constraint coincident L1.end L2.start
  measures "d82" distance of L1.end L4.end
  measures "d83" distance of L1.end L6.end
extrude "Extrude15" cut sketch "Sketch9" against normal blind 12 contours L1 L2 L4 L5 L6 L7 bodies 4
sketch "Sketch10" plane through (0, -52.5, 0) normal (0, -1, 0) x (1, 0, 0)
  line L0 (202.5, 17) -> (202.5, -3)
  line L1 (202.5, -3) -> (332.5, -3)
  line L2 (332.5, -3) -> (332.5, 17)
  line L3 (332.5, 17) -> (202.5, 17)
  line L4 (267.5, 17) -> (267.5, -3) construction
  circle A0 centre (267.5, 7) radius 3
  dimension "d86" = 6
  constraint midpoint L3 L4.start
  constraint midpoint L1 L4.end
  constraint midpoint L4 A0.centre
  measures "d86" diameter of A0
extrude "Extrude16" cut sketch "Sketch10" against normal blind 135 contours A0 bodies 4
sketch "Sketch11" plane through (0, 0, 0) normal (0, 0, 1) x (-1, 0, 0)
  line L0 (-290.5, -42.5) -> (-290.5, -77.5)
  line L1 (-290.5, -77.5) -> (-202.5, -77.5)
  line L2 (-202.5, -77.5) -> (-202.5, 47.5)
  line L3 (-202.5, 47.5) -> (-332.5, 47.5)
  line L4 (-332.5, 47.5) -> (-332.5, -42.5)
  line L5 (-332.5, -42.5) -> (-290.5, -42.5)
  line L6 (-327.5, 47.5) -> (-327.5, -42.5)
  dimension "d89" = -5
extrude "Extrude17" add sketch "Sketch11" along normal blind 17 contours L3 L4 L5 L6 bodies 4
sketch "Sketch12" plane through (332.5, 0, 0) normal (1, 0, 0) x (0, 1, 0)
  line L0 (42.5, -3) -> (42.5, 17)
  line L1 (42.5, 17) -> (-52.5, 17)
  line L2 (-52.5, 17) -> (-52.5, -3)
  line L3 (-52.5, -3) -> (42.5, -3)
  line L4 (-5, 17) -> (-5, -3) construction
  circle A0 centre (-5, 7) radius 3
  dimension "d92" = 6
  constraint midpoint L1 L4.start
  constraint midpoint L3 L4.end
  constraint midpoint L4 A0.centre
  measures "d92" diameter of A0
extrude "Extrude18" cut sketch "Sketch12" against normal blind 5 contours A0 bodies 4
hidden bodies 1
